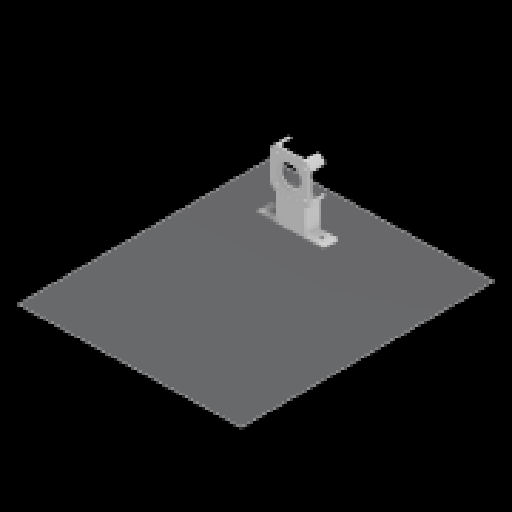
# Autodesk Inventor part: PancakeTopMount
Saved by Autodesk Inventor 2025 (Build 290162000, 162)
## iProperties
Created: 2025-01-12
Part Number: PancakeTopMount
Material: Generic
Document SubType Name: Modeling
Designer: Trevor
Density: 1 g/cm^3
Appearance: Default
Author: Trevor
Autodesk Inventor part; units mm, degrees
ref_plane "YZ Plane" through (0, 0, 0) normal (1, 0, 0) x (0, 1, 0)
ref_plane "XZ Plane" through (0, 0, 0) normal (0, 1, 0) x (-1, 0, 0)
sketch "Sketch1" plane through (0, 0, 0) normal (0, 0, 1) x (1, 0, 0)
  circle A0 centre (-15.5, 15.5) radius 2.85 projected
  line L0 (-20, 16.5858) -> (-16.5858, 20) projected
  line L1 (-20, -16.5858) -> (-20, 16.5858) projected
  line L2 (-16.5858, -20) -> (-20, -16.5858) projected
  line L3 (16.5858, -20) -> (-16.5858, -20) projected
  line L4 (20, -16.5858) -> (16.5858, -20) projected
  line L5 (20, 16.5858) -> (20, -16.5858) projected
  line L6 (16.5858, 20) -> (20, 16.5858) projected
  line L7 (-16.5858, 20) -> (16.5858, 20) projected
  circle A1 centre (15.5, -15.5) radius 1.5 projected
  circle A2 centre (-15.5, 15.5) radius 1.5 projected
  circle A3 centre (-15.5, -15.5) radius 1.5 projected
  circle A4 centre (15.5, 15.5) radius 1.5 projected
  circle A5 centre (0, 0) radius 11 projected
  circle A6 centre (-15.5, 15.5) radius 1.125 projected
  circle A7 centre (-15.5, 15.5) radius 1.225
  circle A8 centre (15.5, 15.5) radius 1.125 projected
  circle A9 centre (15.5, 15.5) radius 1.225
  circle A10 centre (15.5, -15.5) radius 1.5 projected
  arc A11 (14.9226, -16.5) -> (16.0774, -16.5) centre (15.5, -15.5) ccw projected
  arc A12 (16.0774, -16.5) -> (16.6547, -15.5) centre (15.5, -15.5) ccw projected
  arc A13 (16.6547, -15.5) -> (16.0774, -14.5) centre (15.5, -15.5) ccw projected
  arc A14 (16.0774, -14.5) -> (14.9226, -14.5) centre (15.5, -15.5) ccw projected
  arc A15 (14.9226, -14.5) -> (14.3453, -15.5) centre (15.5, -15.5) ccw projected
  arc A16 (14.3453, -15.5) -> (14.9226, -16.5) centre (15.5, -15.5) ccw projected
  circle A17 centre (-15.5, -15.5) radius 1.5 projected
  arc A18 (-16.0774, -16.5) -> (-14.9226, -16.5) centre (-15.5, -15.5) ccw projected
  arc A19 (-14.9226, -16.5) -> (-14.3453, -15.5) centre (-15.5, -15.5) ccw projected
  arc A20 (-14.3453, -15.5) -> (-14.9226, -14.5) centre (-15.5, -15.5) ccw projected
  arc A21 (-14.9226, -14.5) -> (-16.0774, -14.5) centre (-15.5, -15.5) ccw projected
  arc A22 (-16.0774, -14.5) -> (-16.6547, -15.5) centre (-15.5, -15.5) ccw projected
  arc A23 (-16.6547, -15.5) -> (-16.0774, -16.5) centre (-15.5, -15.5) ccw projected
  arc A24 (14.8726, -14.4134) -> (14.2453, -15.5) centre (15.5, -15.5) ccw
  arc A25 (16.1274, -14.4134) -> (14.8726, -14.4134) centre (15.5, -15.5) ccw
  arc A26 (16.7547, -15.5) -> (16.1274, -14.4134) centre (15.5, -15.5) ccw
  arc A27 (16.1274, -16.5866) -> (16.7547, -15.5) centre (15.5, -15.5) ccw
  arc A28 (14.8726, -16.5866) -> (16.1274, -16.5866) centre (15.5, -15.5) ccw
  arc A29 (14.2453, -15.5) -> (14.8726, -16.5866) centre (15.5, -15.5) ccw
  arc A30 (-16.1274, -14.4134) -> (-16.7547, -15.5) centre (-15.5, -15.5) ccw
  arc A31 (-14.8726, -14.4134) -> (-16.1274, -14.4134) centre (-15.5, -15.5) ccw
  arc A32 (-14.2453, -15.5) -> (-14.8726, -14.4134) centre (-15.5, -15.5) ccw
  arc A33 (-14.8726, -16.5866) -> (-14.2453, -15.5) centre (-15.5, -15.5) ccw
  arc A34 (-16.1274, -16.5866) -> (-14.8726, -16.5866) centre (-15.5, -15.5) ccw
  arc A35 (-16.7547, -15.5) -> (-16.1274, -16.5866) centre (-15.5, -15.5) ccw
  circle A36 centre (0, 0) radius 11.1
  line L8 (10, 21) -> (16.5858, 21) projected
  line L9 (17.2929, 20.7071) -> (20.7071, 17.2929) projected
  line L10 (16.5858, 21) -> (16.5858, 20) projected
  arc A37 (17.2929, 20.7071) -> (16.5858, 21) centre (16.5858, 20) ccw projected
  line L11 (-10, 21) -> (10, 21) projected
  line L12 (-16.5858, 21) -> (-10, 21) projected
  line L13 (-20.7071, 17.2929) -> (-17.2929, 20.7071) projected
  arc A38 (-16.5858, 21) -> (-17.2929, 20.7071) centre (-16.5858, 20) ccw projected
  line L14 (-21, 10) -> (-21, 16.5858) projected
  arc A39 (-20.7071, 17.2929) -> (-21, 16.5858) centre (-20, 16.5858) ccw projected
  line L15 (-21, -10) -> (-21, 10) projected
  arc A40 (21, 16.5858) -> (20.7071, 17.2929) centre (20, 16.5858) ccw projected
  line L16 (21, 16.5858) -> (21, 10) projected
  line L17 (21, 10) -> (21, -10) projected
  line L18 (21, -10) -> (21, -16.5858) projected
  arc A41 (20.7071, -17.2929) -> (21, -16.5858) centre (20, -16.5858) ccw projected
  line L19 (21, -16.5858) -> (21, -14.1716) projected
  line L20 (21, -14.1716) -> (14.1716, -21) projected
  line L21 (14.1716, -21) -> (16.5858, -21) projected
  arc A42 (16.5858, -21) -> (17.2929, -20.7071) centre (16.5858, -20) ccw projected
  line L22 (17.2929, -20.7071) -> (20.7071, -17.2929) projected
  line L23 (21, -4) -> (16, -4) projected
  line L24 (16, -4) -> (16, 4) projected
  line L25 (16, 4) -> (21, 4) projected
  line L26 (21, 14.1716) -> (21, 4) projected
  line L27 (21, 14.1716) -> (14.1716, 21) projected
  line L28 (-14.1716, 21) -> (14.1716, 21) projected
  line L29 (-14.1716, 21) -> (-21, 14.1716) projected
  line L30 (-21, -14.1716) -> (-21, 14.1716) projected
  line L31 (-21, -14.1716) -> (-14.1716, -21) projected
  line L32 (14.1716, -21) -> (-14.1716, -21) projected
  line L33 (14.1716, -21) -> (21, -14.1716) projected
  line L34 (21, -4) -> (21, -14.1716) projected
  circle A43 centre (15.5, -15.5) radius 1.5 projected
  circle A44 centre (-15.5, 15.5) radius 1.5 projected
  circle A45 centre (15.5, 15.5) radius 1.5 projected
  circle A46 centre (-15.5, -15.5) radius 1.5 projected
  circle A47 centre (0, 0) radius 4 projected
  arc A48 (-21, -16.5858) -> (-20.7071, -17.2929) centre (-20, -16.5858) ccw projected
  line L35 (-20.7071, -17.2929) -> (-17.2929, -20.7071) projected
  arc A49 (-17.2929, -20.7071) -> (-16.5858, -21) centre (-16.5858, -20) ccw projected
  line L36 (-16.5858, -21) -> (-14.1716, -21) projected
  line L37 (-14.1716, -21) -> (-21, -14.1716) projected
  line L38 (-21, -14.1716) -> (-21, -16.5858) projected
  point P0 (0, 0)
  dimension "d0" = 0.1
  dimension "d1" = 0.1
  dimension "d2" = 0.1
  dimension "d3" = 0.1
  dimension "d6" = 0.1
  constraints: 24 point on circle, 15 centre point, 10 other
  measures "d0" radial gap between concentric circles of A6 A7
  measures "d1" radial gap between concentric circles of A8 A9
  measures "d2" radial gap between concentric circles of A15 A24
  measures "d3" radial gap between concentric circles of A22 A30
  measures "d6" radial gap between concentric circles of A5 A36
extrude "Extrusion1" add sketch "Sketch1" along normal blind 2 contours A0 | L1 L29 L14 A39 L13 A38 L12 L7 L0 | L0 L7 L29 L1 | L29 L7 L27 L5 L25 L24 L23 L20 L3 L31 L1 | L1 L31 L30 L15 L14 L29 | L29 L12 L11 L8 L27 L7 | L31 L3 L2 L1 | L1 L2 L3 L31 L36 A49 L35 A48 L38 | L27 L8 L10 L7 | L7 L6 L5 L27 | L3 L20 L32 L31 | L10 A37 L9 A40 L16 L27 L5 L6 | L27 L16 L17 L25 L5 | L20 L5 L4 L3 | L3 L4 L5 L20 L18 A41 L22 A42 L21 | L25 L17 L23 L5 | L5 L23 L24 L25 | L5 L23 L17 L18 L20 | A2
sketch "Sketch2" plane through (0, 0, 2) normal (0, 0, 1) x (1, 0, 0)
  line L0 (16.5858, 21) -> (-16.5858, 21) projected
  line L1 (16.5858, 21) -> (-16.5858, 21)
  line L2 (-21, 16.5858) -> (-21, -16.5858) projected
  line L3 (-23, -16.2697) -> (-21, -16.2697)
  line L4 (-21, -16.2697) -> (-21, 16.5858)
  line L5 (-16.5858, -21) -> (16.5858, -21) projected
  line L6 (-16.5858, -21) -> (16.5858, -21)
  line L7 (21, -16.5858) -> (21, 16.5858) projected
  line L8 (21, -16.2697) -> (21, 16.5858)
  line L9 (17.2929, 20.7071) -> (20.7071, 17.2929) projected
  arc A0 (17.2929, 20.7071) -> (16.5858, 21) centre (16.5858, 20) ccw projected
  arc A1 (21, 16.5858) -> (20.7071, 17.2929) centre (20, 16.5858) ccw projected
  arc A2 (-16.5858, 21) -> (-17.2929, 20.7071) centre (-16.5858, 20) ccw projected
  line L10 (-20.7071, 17.2929) -> (-17.2929, 20.7071) projected
  arc A3 (-20.7071, 17.2929) -> (-21, 16.5858) centre (-20, 16.5858) ccw projected
  arc A4 (-21, -16.5858) -> (-20.7071, -17.2929) centre (-20, -16.5858) ccw projected
  line L11 (-17.2929, -20.7071) -> (-20.7071, -17.2929) projected
  arc A5 (-17.2929, -20.7071) -> (-16.5858, -21) centre (-16.5858, -20) ccw projected
  arc A6 (16.5858, -21) -> (17.2929, -20.7071) centre (16.5858, -20) ccw projected
  line L12 (20.7071, -17.2929) -> (17.2929, -20.7071) projected
  arc A7 (20.7071, -17.2929) -> (21, -16.5858) centre (20, -16.5858) ccw projected
  line L13 (-16.5858, 21.1) -> (16.5858, 21.1)
  arc A8 (17.3636, 20.7778) -> (16.5858, 21.1) centre (16.5858, 20) ccw
  line L14 (17.3636, 20.7778) -> (20.7778, 17.3636)
  arc A9 (21.1, 16.5858) -> (20.7778, 17.3636) centre (20, 16.5858) ccw
  line L15 (21.1, 16.5858) -> (21.1, -16.5858)
  arc A10 (20.7778, -17.3636) -> (21.1, -16.5858) centre (20, -16.5858) ccw
  line L16 (20.7778, -17.3636) -> (17.3636, -20.7778)
  arc A11 (16.5858, -21.1) -> (17.3636, -20.7778) centre (16.5858, -20) ccw
  line L17 (16.5858, -21.1) -> (-16.5858, -21.1)
  arc A12 (-17.3636, -20.7778) -> (-16.5858, -21.1) centre (-16.5858, -20) ccw
  line L18 (-17.3636, -20.7778) -> (-20.7778, -17.3636)
  arc A13 (-21.1, -16.5858) -> (-20.7778, -17.3636) centre (-20, -16.5858) ccw
  line L19 (-21.1, -16.5858) -> (-21.1, 16.5858)
  arc A14 (-20.7778, 17.3636) -> (-21.1, 16.5858) centre (-20, 16.5858) ccw
  line L20 (-20.7778, 17.3636) -> (-17.3636, 20.7778)
  arc A15 (-16.5858, 21.1) -> (-17.3636, 20.7778) centre (-16.5858, 20) ccw
  line L21 (16.5858, 22.1) -> (-16.5858, 22.1)
  arc A16 (-16.5858, 22.1) -> (-18.0707, 21.4849) centre (-16.5858, 20) ccw
  line L22 (-18.0707, 21.4849) -> (-21.4849, 18.0707)
  arc A17 (-21.4849, 18.0707) -> (-22.1, 16.5858) centre (-20, 16.5858) ccw
  line L23 (-22.1, 16.5858) -> (-22.1, -16.5858)
  arc A18 (-22.1, -16.5858) -> (-21.4849, -18.0707) centre (-20, -16.5858) ccw
  line L24 (-21.4849, -18.0707) -> (-18.0707, -21.4849)
  arc A19 (-18.0707, -21.4849) -> (-16.5858, -22.1) centre (-16.5858, -20) ccw
  line L25 (-16.5858, -22.1) -> (16.5858, -22.1)
  arc A20 (16.5858, -22.1) -> (18.0707, -21.4849) centre (16.5858, -20) ccw
  line L26 (18.0707, -21.4849) -> (21.4849, -18.0707)
  arc A21 (21.4849, -18.0707) -> (22.1, -16.5858) centre (20, -16.5858) ccw
  line L27 (22.1, -16.5858) -> (22.1, 16.5858)
  arc A22 (22.1, 16.5858) -> (21.4849, 18.0707) centre (20, 16.5858) ccw
  line L28 (21.4849, 18.0707) -> (18.0707, 21.4849)
  arc A23 (18.0707, 21.4849) -> (16.5858, 22.1) centre (16.5858, 20) ccw
  point P0 (0, 0)
  dimension "d8" = 2
  dimension "d11" = 0.1
  dimension "d12" = 1
  constraints: 42 end point, 32 point on circle, 16 centre point, 2 horizontal, 30 other
  measures "d8" distance of L3.end L3.start
  measures "d11" distance between parallel lines of L0 L13
  measures "d12" distance between parallel lines of L13 L21
ref_plane "Work Plane1" through (-21.979, -21.979, -14) normal (0, 0, 1) x (1, 0, 0)
extrude "Extrusion2" add sketch "Sketch2" against normal up to surface (16 mm away) contours A23 L28 A22 L27 A21 L26 A20 L25 A19 L24 A18 L23 A17 L22 A16 L21
sketch "Sketch3" plane through (0, 0, 2) normal (0, 0, 1) x (1, 0, 0)
  line L0 (-16.5858, -22.1) -> (16.5858, -22.1) projected
  line L1 (-66.059, -53.6381) -> (148.6826, -48.6301) projected
  line L2 (16.5858, -22.1) -> (16.5858, -51.7107)
  line L3 (-16.5858, -22.1) -> (-16.5858, -52.4843)
  point P0 (0, 0)
  constraints: 4 end point, 2 point on line, 1 parallel, 1 vertical
extrude "Extrusion3" add sketch "Sketch3" against normal up to surface (16 mm away)
ref_plane "Work Plane2" through (31.3145, -51.3672, 81.375) normal (-0.0233148, 0.9997282, 0) x (0, 0, -1)
sketch "Sketch4" plane through (31.3145, -51.3672, 81.375) normal (-0.0233148, 0.9997282, 0) x (0, 0, -1)
  line L0 (79.375, 14.7328) -> (95.375, 14.7328) projected
  line L1 (79.375, 47.9134) -> (95.375, 47.9134) projected
  line L2 (95.375, 47.9134) -> (79.8386, 47.9134)
  line L3 (79.375, 52.5891) -> (95.375, 52.5891) projected
  line L4 (95.375, 14.7328) -> (95.375, 47.9134) projected
  line L5 (79.375, 47.9134) -> (79.375, 14.7328) projected
  line L6 (79.375, 14.7328) -> (95.375, 14.7328)
  line L7 (95.375, 14.7328) -> (79.375, 14.7328)
  line L8 (79.375, 14.7328) -> (79.375, -5.2672)
  line L9 (79.375, -5.2672) -> (95.375, -5.2672)
  line L10 (95.375, -5.2672) -> (95.375, 14.7328)
  line L11 (95.375, 47.9134) -> (95.375, 47.2049) projected
  line L12 (95.375, 47.9134) -> (79.375, 47.9134)
  line L13 (79.375, 47.9134) -> (79.375, 67.9134)
  line L14 (79.375, 67.9134) -> (95.375, 67.9134)
  line L15 (95.375, 67.9134) -> (95.375, 47.9134)
  circle A0 centre (87.375, 4.7328) radius 2.5
  circle A1 centre (87.375, 57.9134) radius 2.5
  point P0 (81.375, 30.1084)
  point P1 (79.375, 47.9134)
  dimension "d23" = 20
  dimension "d24" = 20
  dimension "d25" = 5
  dimension "d26" = 5
  dimension "d27" = 10
  dimension "d28" = 10
  constraints: 20 end point, 4 horizontal, 4 parallel, 2 centre point, 2 perpendicular, 1 point on line
  measures "d23" distance of L8.end L7.end
  measures "d24" distance of L12.end L13.end
  measures "d25" diameter of A0
  measures "d26" diameter of A1
  measures "d27" distance from line of L14 A1.centre
  measures "d28" distance from line of L9 A0.centre
extrude "Extrusion4" add sketch "Sketch4" along normal blind 2 contours L0 L10 L9 L8 | L13 L3 L15 L1 | L13 L14 L15 L3
sketch "Sketch5" plane through (-16.5858, 22.1, 2) normal (0, 1, 0) x (1, 0, 0)
  line L0 (0, 0) -> (33.1716, 0) projected
  line L1 (16.5858, 0) -> (16.5858, 2)
  line L2 (16.5858, 2) -> (30.5858, 2)
  line L3 (30.5858, 2) -> (30.5858, 16)
  line L4 (30.5858, 16) -> (16.5858, 16)
  line L5 (16.5858, 16) -> (16.5858, 2)
  line L6 (16.5858, 2) -> (2.5858, 2)
  line L7 (2.5858, 2) -> (2.5858, 16)
  line L8 (2.5858, 16) -> (16.5858, 16)
  line L9 (16.5858, 16) -> (16.5858, 2)
  dimension "d29" = 14
  dimension "d30" = 14
  dimension "d31" = 14
  dimension "d32" = 14
  constraints: 18 end point, 4 parallel, 2 horizontal, 2 perpendicular, 1 midpoint, 1 vertical
  measures "d29" distance of L4.end L3.end
  measures "d30" distance of L3.end L2.end
  measures "d31" distance of L7.end L8.end
  measures "d32" distance of L6.end L7.end
extrude "Extrusion5" cut sketch "Sketch5" against normal up to surface (1 mm away)
sketch "Sketch6" plane through (-22.1, -16.5858, 2) normal (-1, 0, 0) x (0, 0, 1)
  line L0 (-2, 16.5858) -> (-16, 16.5858)
  line L1 (-16, 0) -> (-16, 33.1716) projected
  line L2 (-2, 16.5858) -> (-16, 16.5858)
  line L3 (-16, 16.5858) -> (-16, 30.5858)
  line L4 (-16, 30.5858) -> (-2, 30.5858)
  line L5 (-2, 30.5858) -> (-2, 16.5858)
  line L6 (-2, 16.5858) -> (-16, 16.5858)
  line L7 (-16, 16.5858) -> (-16, 2.5858)
  line L8 (-16, 2.5858) -> (-2, 2.5858)
  line L9 (-2, 2.5858) -> (-2, 16.5858)
  dimension "d35" = 14
  dimension "d36" = 14
  dimension "d37" = 14
  constraints: 18 end point, 4 parallel, 2 horizontal, 2 perpendicular, 1 midpoint, 1 point on line
  measures "d35" distance of L3.end L4.end
  measures "d36" distance of L2.end L3.end
  measures "d37" distance of L7.end L6.end
extrude "Extrusion6" cut sketch "Sketch6" against normal up to surface (1 mm away)
sketch "Sketch7" plane through (22.1, -16.5858, 2) normal (1, 0, 0) x (0, 0, -1)
  line L0 (16, 33.1716) -> (16, 0) projected
  line L1 (16, 16.5858) -> (0, 16.5858)
  line L2 (0, 0) -> (0, 33.1716) projected
  line L3 (16, 16.5858) -> (2, 16.5858)
  line L4 (2, 16.5858) -> (2, 30.5858)
  line L5 (2, 30.5858) -> (16, 30.5858)
  line L6 (16, 30.5858) -> (16, 16.5858)
  line L7 (16, 16.5858) -> (2, 16.5858)
  line L8 (2, 16.5858) -> (2, 2.5858)
  line L9 (2, 2.5858) -> (16, 2.5858)
  line L10 (16, 2.5858) -> (16, 16.5858)
  point P0 (2, 16.5858)
  point P1 (2, 16.5858)
  dimension "d40" = 14
  dimension "d41" = 14
  dimension "d42" = 14
  dimension "d43" = 14
  constraints: 18 end point, 4 parallel, 2 horizontal, 2 midpoint, 2 perpendicular
  measures "d40" distance of L4.end L5.end
  measures "d41" distance of L3.end L4.end
  measures "d42" distance of L9.end L8.end
  measures "d43" distance of L8.end L7.end
extrude "Extrusion7" cut sketch "Sketch7" against normal up to surface (1 mm away)
equation "\"d1\" = d0"
equation "\"d2\" = d0"
equation "\"d3\" = d0"
body "Solid1"
